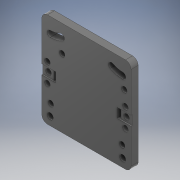
# Autodesk Inventor part: x carraige plate new
Saved by Autodesk Inventor 2020.2 (Build 242310000, 310)
## iProperties
Created: 2019-11-18
Part Number: x carraige plate new
Material: PMMA Plastic
Document SubType Name: Modeling
Designer: Richard Hall
Density: 1.188 g/cm^3
Appearance: Smooth - Black
Author: Richard Hall
Autodesk Inventor part; units mm, degrees
ref_plane "YZ Plane" through (0, 0, 0) normal (1, 0, 0) x (0, 1, 0)
ref_plane "XZ Plane" through (0, 0, 0) normal (0, 1, 0) x (-1, 0, 0)
ref_plane "XY Plane" through (0, 0, 0) normal (0, 0, 1) x (1, 0, 0)
sketch "Sketch1" plane through (0, 0, 0) normal (0, 0, 1) x (1, 0, 0)
  line L0 (-40, -42.5) -> (40, -42.5)
  line L1 (40, -42.5) -> (40, 42.5)
  line L2 (40, 42.5) -> (-40, 42.5)
  line L3 (-40, 42.5) -> (-40, -42.5)
  line L4 (-40, -42.5) -> (40, 42.5) construction
  line L5 (40, -42.5) -> (-40, 42.5) construction
  line L6 (-28.7479, 32.175) -> (28.7479, 32.175) construction
  line L7 (28.7479, 32.175) -> (28.7479, -32.175) construction
  line L8 (28.7479, -32.175) -> (-28.7479, -32.175) construction
  line L9 (-28.7479, -32.175) -> (-28.7479, 32.175) construction
  line L10 (-28.7479, 32.175) -> (28.7479, -32.175) construction
  line L11 (28.7479, 32.175) -> (-28.7479, -32.175) construction
  circle A0 centre (28.7479, -32.175) radius 2.5 construction
  circle A1 centre (-28.7479, -32.175) radius 2.5 construction
  arc A2 (-28.7479, 32.175) -> (-13.7479, 34.175) centre (-28.7479, 89.425) ccw construction
  arc A3 (-28.7479, 29.675) -> (-13.0929, 31.7623) centre (-28.7479, 89.425) ccw construction
  arc A4 (-28.7479, 34.675) -> (-14.403, 36.5877) centre (-28.7479, 89.425) ccw construction
  arc A5 (-28.7479, 34.675) -> (-28.7479, 29.675) centre (-28.7479, 32.175) ccw construction
  arc A6 (-13.0929, 31.7623) -> (-14.403, 36.5877) centre (-13.7479, 34.175) ccw construction
  point P0 (0, 0)
  dimension "d0" = 80
  dimension "d1" = 64.35
  dimension "d2" = 5
  dimension "d3" = 5
  dimension "d4" = 5
  dimension "d5" = 2
  dimension "d6" = 15
  dimension "d7" = 85
  constraints: 24 end point, 10 point on circle, 7 centre point, 5 tangent, 4 midpoint, 4 parallel, 2 coincident, 2 horizontal, 2 perpendicular
  measures "d0" distance of L2.end L1.end
  measures "d1" distance of L6.end L7.end
  measures "d2" diameter of A0
  measures "d3" diameter of A1
  measures "d4" diameter of A6
  measures "d5" distance from line of L6 A2.end
  measures "d6" horizontal distance of L6.start A2.end
  measures "d7" distance of L0.end L1.end
extrude "Extrusion1" add sketch "Sketch1" along normal mid plane 6.35
sketch "Sketch2" plane through (0, 0, 3.175) normal (0, 0, 1) x (1, 0, 0)
  line L0 (-40, -42.5) -> (40, -42.5) projected
  line L1 (-40, 42.5) -> (-40, -42.5) projected
  line L2 (40, -42.5) -> (40, 42.5) projected
  point P0 (0, 0)
  point P1 (-32.5, -35)
  point P2 (32.5, -35)
  dimension "d11" = 7.5
  dimension "d12" = 7.5
  dimension "d13" = 7.5
  constraints: 1 horizontal alignment
  measures "d11" distance from line of L0 point (-32.5, -35)
  measures "d12" distance from line of L1 point (-32.5, -35)
  measures "d13" distance from line of L2 point (32.5, -35)
hole "Hole1" at (-32.5, -35, 3.175) at (32.5, -35, 3.175) direction (0, 0, -1) diameter 5.5 end through all start extended yes clearance for "Flat Head Machine Screw" size "M5" standard "Ansi Metric M Profile"
sketch "Sketch3" plane through (0, 0, 3.175) normal (0, 0, 1) x (1, 0, 0)
  circle A0 centre (-32.5, -35) radius 2.75 projected
  circle A1 centre (32.5, -35) radius 2.75 projected
  arc A2 (-32.5, 29) -> (-22.5, 31.5) centre (-32.5, 50.25) ccw construction
  arc A3 (-32.5, 26.25) -> (-21.2059, 29.0735) centre (-32.5, 50.25) ccw
  arc A4 (-32.5, 31.75) -> (-23.7941, 33.9265) centre (-32.5, 50.25) ccw
  arc A5 (-32.5, 31.75) -> (-32.5, 26.25) centre (-32.5, 29) ccw
  arc A6 (-21.2059, 29.0735) -> (-23.7941, 33.9265) centre (-22.5, 31.5) ccw
  line L0 (0, 0) -> (0, 8.7533)
  arc A7 (22.5, 31.5) -> (32.5, 29) centre (32.5, 50.25) ccw construction
  arc A8 (21.2059, 29.0735) -> (32.5, 26.25) centre (32.5, 50.25) ccw
  arc A9 (23.7941, 33.9265) -> (32.5, 31.75) centre (32.5, 50.25) ccw
  arc A10 (32.5, 26.25) -> (32.5, 31.75) centre (32.5, 29) ccw
  arc A11 (23.7941, 33.9265) -> (21.2059, 29.0735) centre (22.5, 31.5) ccw
  dimension "d21" = 64
  dimension "d22" = 2.5
  dimension "d23" = 10
  dimension "d24" = 2.75
  constraints: 20 point on circle, 10 centre point, 7 symmetric about line, 4 tangent, 2 end point, 2 vertical alignment, 1 vertical, 5 other
  measures "d21" distance of A0.centre A2.start
  measures "d22" vertical distance of A2.start A2.end
  measures "d23" horizontal distance of A2.end A2.start
  measures "d24" radius of A6
extrude "Extrusion2" cut sketch "Sketch3" against normal blind 10 contours A5 A4 A6 A3 | A11 A9 A10 A8
fillet "Fillet1" radius 5 4 edges at (-40, 42.5, 0) (-40, -42.5, 0) (40, 42.5, 0) (40, -42.5, 0)
sketch "Sketch5" plane through (0, 0, 3.175) normal (0, 0, 1) x (1, 0, 0)
  line L0 (-35, 1.95) -> (-32.5, 1.95)
  line L1 (-32.5, 1.95) -> (-32.5, -6.55)
  line L2 (-32.5, -6.55) -> (-35, -6.55)
  line L3 (-35, -6.55) -> (-35, 1.95)
  line L4 (-35, 1.95) -> (-32.5, -6.55) construction
  line L5 (-32.5, 1.95) -> (-35, -6.55) construction
  line L6 (-35, -42.5) -> (35, -42.5) projected
  line L7 (-40, 37.5) -> (-40, -37.5) projected
  line L8 (0, 0) -> (0, 7.9941)
  line L9 (35, 1.95) -> (32.5, 1.95)
  line L10 (32.5, 1.95) -> (32.5, -6.55)
  line L11 (32.5, -6.55) -> (35, -6.55)
  line L12 (35, -6.55) -> (35, 1.95)
  line L13 (35, 1.95) -> (32.5, -6.55) construction
  line L14 (32.5, 1.95) -> (35, -6.55) construction
  line L15 (-38, -2.3) -> (-40, -3.4547)
  line L16 (-40, -3.4547) -> (-40, -1.1453)
  line L17 (-40, -1.1453) -> (-38, -2.3)
  line L18 (38, -2.3) -> (40, -3.4547)
  line L19 (40, -3.4547) -> (40, -1.1453)
  line L20 (40, -1.1453) -> (38, -2.3)
  line L21 (-30, 1.95) -> (-27.5, 1.95)
  line L22 (-27.5, 1.95) -> (-27.5, -6.55)
  line L23 (-27.5, -6.55) -> (-30, -6.55)
  line L24 (-30, -6.55) -> (-30, 1.95)
  line L25 (-30, 1.95) -> (-27.5, -6.55) construction
  line L26 (-27.5, 1.95) -> (-30, -6.55) construction
  line L27 (30, 1.95) -> (27.5, 1.95)
  line L28 (27.5, 1.95) -> (27.5, -6.55)
  line L29 (27.5, -6.55) -> (30, -6.55)
  line L30 (30, -6.55) -> (30, 1.95)
  line L31 (30, 1.95) -> (27.5, -6.55) construction
  line L32 (27.5, 1.95) -> (30, -6.55) construction
  line L33 (-22.5, 1.95) -> (-20, 1.95)
  line L34 (-20, 1.95) -> (-20, -6.55)
  line L35 (-20, -6.55) -> (-22.5, -6.55)
  line L36 (-22.5, -6.55) -> (-22.5, 1.95)
  line L37 (-22.5, 1.95) -> (-20, -6.55) construction
  line L38 (-20, 1.95) -> (-22.5, -6.55) construction
  line L39 (20, 1.95) -> (22.5, 1.95)
  line L40 (22.5, 1.95) -> (22.5, -6.55)
  line L41 (22.5, -6.55) -> (20, -6.55)
  line L42 (20, -6.55) -> (20, 1.95)
  line L43 (20, 1.95) -> (22.5, -6.55) construction
  line L44 (22.5, 1.95) -> (20, -6.55) construction
  point P0 (-33.75, -2.3)
  point P1 (33.75, -2.3)
  point P2 (-39.3333, -2.3)
  point P3 (-33.75, -2.3)
  point P4 (39.3333, -2.3)
  point P5 (-40, -1.1453)
  point P6 (-28.75, -2.3)
  point P7 (-28.75, -2.3)
  point P8 (-33.75, -2.3)
  point P9 (28.75, -2.3)
  point P10 (28.75, -2.3)
  point P11 (-21.25, -2.3)
  point P12 (21.25, -2.3)
  dimension "d40" = 2.5
  dimension "d41" = 8.5
  dimension "d42" = 40.2
  dimension "d46" = 2
  dimension "d51" = 5
  dimension "d52" = 5
  dimension "d53" = 5
  dimension "d69" = 10
  constraints: 86 end point, 15 midpoint, 15 symmetric about line, 8 parallel, 5 collinear, 4 equal length, 4 horizontal, 4 perpendicular, 2 horizontal alignment, 1 vertical, 7 other
  measures "d40" distance of L1.end L2.end
  measures "d41" distance of L0.end L1.end
  measures "d42" distance from line of L6 point (-33.75, -2.3)
  measures "d46" horizontal distance of L16.end L15.start
  measures "d51" distance between parallel lines of L7 L3
  measures "d52" distance between parallel lines of L36 L22
  measures "d53" distance between parallel lines of L28 L40
  measures "d69" distance between parallel lines of L7 L24
extrude "Extrusion3" cut sketch "Sketch5" against normal blind 10 contours L21 L22 L23 L24 | L30 L29 L28 L27
sketch "Sketch7" plane through (0, 0, 3.175) normal (0, 0, 1) x (1, 0, 0)
  line L0 (30, 1.95) -> (30, -6.55) projected
  line L1 (30, -6.55) -> (27.5, -6.55) projected
  line L2 (27.5, -6.55) -> (27.5, 1.95) projected
  line L3 (27.5, 1.95) -> (30, 1.95) projected
  line L4 (-27.5, 1.95) -> (-27.5, -6.55) projected
  line L5 (-27.5, -6.55) -> (-30, -6.55) projected
  line L6 (-30, -6.55) -> (-30, 1.95) projected
  line L7 (-30, 1.95) -> (-27.5, 1.95) projected
  arc A0 (35, -42.5) -> (40, -37.5) centre (35, -37.5) ccw projected
  line L8 (40, -37.5) -> (40, 37.5) projected
  arc A1 (40, 37.5) -> (35, 42.5) centre (35, 37.5) ccw projected
  line L9 (35, 42.5) -> (-35, 42.5) projected
  arc A2 (-35, 42.5) -> (-40, 37.5) centre (-35, 37.5) ccw projected
  line L10 (-40, 37.5) -> (-40, -37.5) projected
  arc A3 (-40, -37.5) -> (-35, -42.5) centre (-35, -37.5) ccw projected
  line L11 (-35, -42.5) -> (35, -42.5) projected
  arc A4 (23.7941, 33.9265) -> (32.5, 31.75) centre (32.5, 50.25) ccw projected
  arc A5 (32.5, 26.25) -> (32.5, 31.75) centre (32.5, 29) ccw projected
  arc A6 (21.2059, 29.0735) -> (32.5, 26.25) centre (32.5, 50.25) ccw projected
  arc A7 (23.7941, 33.9265) -> (21.2059, 29.0735) centre (22.5, 31.5) ccw projected
  arc A8 (-32.5, 26.25) -> (-21.2059, 29.0735) centre (-32.5, 50.25) ccw projected
  arc A9 (-32.5, 31.75) -> (-32.5, 26.25) centre (-32.5, 29) ccw projected
  arc A10 (-32.5, 31.75) -> (-23.7941, 33.9265) centre (-32.5, 50.25) ccw projected
  arc A11 (-21.2059, 29.0735) -> (-23.7941, 33.9265) centre (-22.5, 31.5) ccw projected
  circle A12 centre (-32.5, -35) radius 2.75 projected
  circle A13 centre (32.5, -35) radius 2.75 projected
  line L12 (-30, 1.95) -> (-27.5, 1.95) projected
  line L13 (-30, 1.95) -> (-40, 1.95)
  line L14 (-40, 1.95) -> (-40, -6.55)
  line L15 (-40, -6.55) -> (-30, -6.55)
  line L16 (-30, -6.55) -> (-30, 1.95)
  line L17 (30, -6.55) -> (30, 1.95) projected
  line L18 (30, 1.95) -> (40, 1.95)
  line L19 (40, 1.95) -> (40, -6.55)
  line L20 (40, -6.55) -> (30, -6.55)
  line L21 (30, -6.55) -> (30, 1.95)
  point P0 (0, 0)
  constraints: 16 end point, 4 collinear, 4 parallel, 2 horizontal, 2 perpendicular
extrude "Extrusion5" cut sketch "Sketch7" against normal blind 1 contours L18 L8 L20 L0 | L13 L6 L15 L10
sketch "Sketch8" plane through (0, 0, 3.175) normal (0, 0, 1) x (1, 0, 0)
  line L0 (-40, 1.95) -> (-30, 1.95) projected
  line L1 (-40, -6.55) -> (-40, 1.95) projected
  line L2 (-30, -6.55) -> (-40, -6.55) projected
  line L3 (-30, 1.95) -> (-30, -6.55) projected
  line L4 (30, 1.95) -> (40, 1.95) projected
  line L5 (30, -6.55) -> (30, 1.95) projected
  line L6 (40, -6.55) -> (30, -6.55) projected
  line L7 (40, 1.95) -> (40, -6.55) projected
  circle A0 centre (-35, -2.3) radius 2.5
  circle A1 centre (35, -2.3) radius 2.5
  point P0 (0, 0)
  point P1 (-35, 1.95)
  point P2 (-30, -2.3)
  point P3 (30, -2.3)
  point P4 (35, 1.95)
  dimension "d56" = 5
  dimension "d57" = 5
  constraints: 4 midpoint, 2 centre point, 2 horizontal alignment, 2 vertical alignment
  measures "d56" diameter of A0
  measures "d57" diameter of A1
extrude "Extrusion6" cut sketch "Sketch8" against normal blind 10 contours A0 | A1
sketch "Sketch9" plane through (0, 0, 3.175) normal (0, 0, 1) x (1, 0, 0)
  circle A0 centre (32.5, -35) radius 2.75 projected
  circle A1 centre (-32.5, -35) radius 2.75 projected
  arc A2 (-32.5, 26.25) -> (-21.2059, 29.0735) centre (-32.5, 50.25) ccw projected
  arc A3 (-32.5, 31.75) -> (-32.5, 26.25) centre (-32.5, 29) ccw projected
  arc A4 (-32.5, 31.75) -> (-23.7941, 33.9265) centre (-32.5, 50.25) ccw projected
  arc A5 (-21.2059, 29.0735) -> (-23.7941, 33.9265) centre (-22.5, 31.5) ccw projected
  arc A6 (23.7941, 33.9265) -> (32.5, 31.75) centre (32.5, 50.25) ccw projected
  arc A7 (32.5, 26.25) -> (32.5, 31.75) centre (32.5, 29) ccw projected
  arc A8 (21.2059, 29.0735) -> (32.5, 26.25) centre (32.5, 50.25) ccw projected
  arc A9 (23.7941, 33.9265) -> (21.2059, 29.0735) centre (22.5, 31.5) ccw projected
  line L0 (27.5, 1.95) -> (40, 1.95) projected
  line L1 (40, 1.95) -> (40, 37.5) projected
  arc A10 (40, 37.5) -> (35, 42.5) centre (35, 37.5) ccw projected
  line L2 (35, 42.5) -> (-35, 42.5) projected
  arc A11 (-35, 42.5) -> (-40, 37.5) centre (-35, 37.5) ccw projected
  line L3 (-40, 37.5) -> (-40, 1.95) projected
  line L4 (-40, 1.95) -> (-27.5, 1.95) projected
  line L5 (-27.5, 1.95) -> (-27.5, -6.55) projected
  line L6 (-27.5, -6.55) -> (-40, -6.55) projected
  line L7 (-40, -6.55) -> (-40, -37.5) projected
  arc A12 (-40, -37.5) -> (-35, -42.5) centre (-35, -37.5) ccw projected
  line L8 (-35, -42.5) -> (35, -42.5) projected
  arc A13 (35, -42.5) -> (40, -37.5) centre (35, -37.5) ccw projected
  line L9 (40, -37.5) -> (40, -6.55) projected
  line L10 (40, -6.55) -> (27.5, -6.55) projected
  line L11 (27.5, -6.55) -> (27.5, 1.95) projected
  circle A14 centre (-35, -2.3) radius 2.5 projected
  circle A15 centre (35, -2.3) radius 2.5 projected
  point P0 (0, 0)
  point P1 (-35, 6.2)
  point P2 (-35, -10.8)
  point P3 (35, -10.8)
  point P4 (35, 6.2)
  dimension "d60" = 17
  dimension "d61" = 8.5
  constraints: 4 vertical alignment, 2 horizontal alignment
  measures "d60" distance of point (-35, -10.8) point (-35, 6.2)
  measures "d61" distance of A14.centre point (-35, 6.2)
hole "Hole3" at (-35, 6.2, 3.175) at (-35, -10.8, 3.175) at (35, -10.8, 3.175) at (35, 6.2, 3.175) direction (0, 0, -1) diameter 5 depth 28.25 tip angle 118 start extended yes
sketch "Sketch10" plane through (0, 0, 3.175) normal (0, 0, 1) x (1, 0, 0)
  line L0 (-20, 20) -> (20, 20) construction
  line L1 (20, 20) -> (20, -20) construction
  line L2 (20, -20) -> (-20, -20) construction
  line L3 (-20, -20) -> (-20, 20) construction
  line L4 (-20, 20) -> (20, -20) construction
  line L5 (20, 20) -> (-20, -20) construction
  line L6 (-10, 31.25) -> (10, 31.25) construction
  line L7 (35, 42.5) -> (-35, 42.5) construction
  line L8 (-10, -31.25) -> (10, -31.25) construction
  line L9 (-32, 18.9) -> (32, 18.9) construction
  line L10 (32, 18.9) -> (32, -24.9) construction
  line L11 (32, -24.9) -> (-32, -24.9) construction
  line L12 (-32, -24.9) -> (-32, 18.9) construction
  line L13 (-32, 18.9) -> (32, -24.9) construction
  line L14 (32, 18.9) -> (-32, -24.9) construction
  point P0 (0, 0)
  point P1 (0, 31.25)
  point P2 (0, 0)
  point P3 (0, -31.25)
  point P4 (0, 0)
  point P5 (0, -3)
  point P6 (0, -3)
  point P7 (34, 18.9)
  point P8 (-21.8, 18.9)
  dimension "d70" = 40
  dimension "d71" = 40
  dimension "d72" = 20
  dimension "d73" = 11.25
  dimension "d74" = 11.25
  dimension "d75" = 11.25
  dimension "d83" = 64
  dimension "d84" = 43.8
  dimension "d85" = 24.9
  dimension "d86" = 2
  dimension "d87" = 10.2
  constraints: 28 end point, 10 coincident, 9 midpoint, 5 parallel, 4 horizontal, 3 vertical alignment, 2 perpendicular, 2 point on line
  measures "d70" distance of L1.end L2.end
  measures "d71" distance of L0.end L1.end
  measures "d72" distance of L6.start L6.end
  measures "d73" distance between parallel lines of L0 L6
  measures "d74" distance between parallel lines of L6 L7
  measures "d75" distance between parallel lines of L8 L2
  measures "d83" distance of L10.end L11.end
  measures "d84" distance of L9.end L10.end
  measures "d85" distance from line of L11 point (0, 0)
  measures "d86" distance from line of L10 point (34, 18.9)
  measures "d87" distance from line of L12 point (-21.8, 18.9)
hole "Hole4" at (-21.8, 18.9, 3.175) at (34, 18.9, 3.175) at (32, -24.9, 3.175) at (-32, -24.9, 3.175) direction (0, 0, -1) diameter 5 end through all start extended yes
sketch "Sketch11" plane through (0, 0, 3.175) normal (0, 0, 1) x (1, 0, 0)
  line L0 (-29.6544, 25.4909) -> (-13.6801, 25.4909)
  line L1 (-13.6801, 25.4909) -> (-13.6801, 10.7062)
  line L2 (-13.6801, 10.7062) -> (-29.6544, 10.7062)
  line L3 (-29.6544, 10.7062) -> (-29.6544, 25.4909)
  point P0 (0, 0)
  constraints: 8 end point, 2 parallel, 1 horizontal, 1 perpendicular
extrude "Extrusion7" [suppressed]
equation "\"d52\" = d51"
equation "\"d53\" = d52"
equation "\"d61\" = 0.5 * d60"
equation "\"d74\" = d73"
equation "\"d75\" = d73"
body "Solid1"
